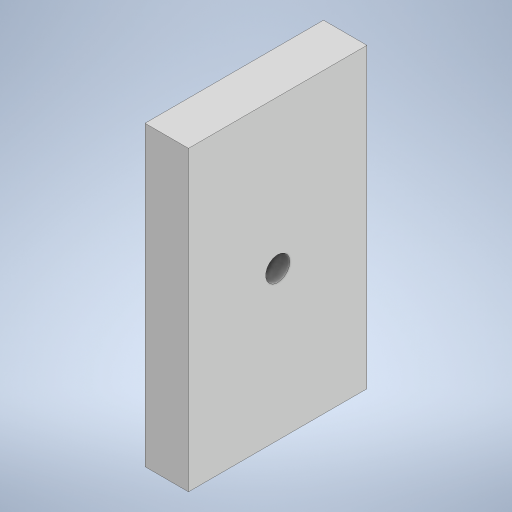
# Autodesk Inventor part: Part1
Saved by Autodesk Inventor 2023 (Build 270158000, 158)
## iProperties
Created: 2024-08-09
Part Number: Part1
Material: Generic
Document SubType Name: Modeling
Designer: sebas
Density: 1 g/cm^3
Appearance: Default
Author: sebas
Autodesk Inventor part; units mm, degrees
ref_plane "YZ Plane" through (0, 0, 0) normal (1, 0, 0) x (0, 1, 0)
ref_plane "XZ Plane" through (0, 0, 0) normal (0, 1, 0) x (-1, 0, 0)
ref_plane "XY Plane" through (0, 0, 0) normal (0, 0, 1) x (1, 0, 0)
sketch "Sketch1" plane through (0, 0, 0) normal (0, 1, 0) x (-1, 0, 0)
  line L0 (0, 0) -> (9.5, 0)
  line L1 (9.5, 0) -> (9.5, -39)
  line L2 (9.5, -39) -> (0, -39)
  line L3 (0, -39) -> (0, 0)
  dimension "d0" = 9.5
  dimension "d2" = 39
  constraints: 8 end point, 2 perpendicular, 1 horizontal, 1 vertical
  measures "d0" distance of L0.start L0.end
  measures "d2" distance of L0.end L1.end
extrude "Extrusion1" add sketch "Sketch1" along normal blind 65
sketch "Sketch2" plane through (0, 0, 0) normal (1, 0, 0) x (0, 0, -1)
  line L0 (39, 65) -> (0, 65) projected
  line L1 (0, 65) -> (39, 0)
  circle A0 centre (19.5, 32.5) radius 2.65
  point P0 (0, 0)
  dimension "d5" = 5.3
  constraints: 2 end point, 1 centre point, 1 midpoint
  measures "d5" diameter of A0
extrude "Extrusion2" cut sketch "Sketch2" against normal through all
body "Solid1"
